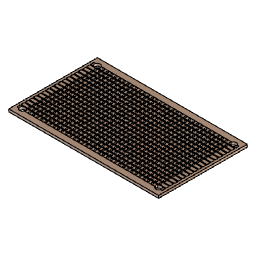
head (Autodesk Fusion 360 archive; units mm, degrees)
design "Veroboard v6"
Autodesk Fusion 360 part; units mm, degrees
sketch "Sketch2" plane through (0, 0, 0) normal (0, 0, 1) x (1, 0, 0) in component "55x93 Tayda Veroboard"
  line L0 (46.5, -27.5) -> (-46.5, -27.5)
  line L1 (-46.5, -27.5) -> (-46.5, 27.5)
  line L2 (-46.5, 27.5) -> (46.5, 27.5)
  line L3 (46.5, 27.5) -> (46.5, -27.5)
  line L4 (46.5, -27.5) -> (-46.5, 27.5) construction
  line L5 (-46.5, -27.5) -> (46.5, 27.5) construction
  line L6 (45, 1) -> (-45, 1)
  line L7 (-45, 1) -> (-45, -1)
  line L8 (-45, -1) -> (45, -1)
  line L9 (45, -1) -> (45, 1)
  line L10 (45, 1) -> (-45, -1) construction
  line L11 (-45, 1) -> (45, -1) construction
  line L12 (45, -21.86) -> (-45, -21.86)
  line L13 (-45, -23.86) -> (45, -23.86)
  line L14 (45, -23.86) -> (45, -21.86)
  line L15 (-45, -21.86) -> (-45, -23.86)
  line L16 (45, -19.32) -> (-45, -19.32)
  line L17 (-45, -21.32) -> (45, -21.32)
  line L18 (45, -21.32) -> (45, -19.32)
  line L19 (-45, -19.32) -> (-45, -21.32)
  line L20 (45, -16.78) -> (-45, -16.78)
  line L21 (-45, -18.78) -> (45, -18.78)
  line L22 (45, -18.78) -> (45, -16.78)
  line L23 (-45, -16.78) -> (-45, -18.78)
  line L24 (45, -14.24) -> (-45, -14.24)
  line L25 (-45, -16.24) -> (45, -16.24)
  line L26 (45, -16.24) -> (45, -14.24)
  line L27 (-45, -14.24) -> (-45, -16.24)
  line L28 (45, -11.7) -> (-45, -11.7)
  line L29 (-45, -13.7) -> (45, -13.7)
  line L30 (45, -13.7) -> (45, -11.7)
  line L31 (-45, -11.7) -> (-45, -13.7)
  line L32 (45, -9.16) -> (-45, -9.16)
  line L33 (-45, -11.16) -> (45, -11.16)
  line L34 (45, -11.16) -> (45, -9.16)
  line L35 (-45, -9.16) -> (-45, -11.16)
  line L36 (45, -6.62) -> (-45, -6.62)
  line L37 (-45, -8.62) -> (45, -8.62)
  line L38 (45, -8.62) -> (45, -6.62)
  line L39 (-45, -6.62) -> (-45, -8.62)
  line L40 (45, -4.08) -> (-45, -4.08)
  line L41 (-45, -6.08) -> (45, -6.08)
  line L42 (45, -6.08) -> (45, -4.08)
  line L43 (-45, -4.08) -> (-45, -6.08)
  line L44 (45, -1.54) -> (-45, -1.54)
  line L45 (-45, -3.54) -> (45, -3.54)
  line L46 (45, -3.54) -> (45, -1.54)
  line L47 (-45, -1.54) -> (-45, -3.54)
  line L48 (45, 3.54) -> (-45, 3.54)
  line L49 (-45, 1.54) -> (45, 1.54)
  line L50 (45, 1.54) -> (45, 3.54)
  line L51 (-45, 3.54) -> (-45, 1.54)
  line L52 (45, 6.08) -> (-45, 6.08)
  line L53 (-45, 4.08) -> (45, 4.08)
  line L54 (45, 4.08) -> (45, 6.08)
  line L55 (-45, 6.08) -> (-45, 4.08)
  line L56 (45, 8.62) -> (-45, 8.62)
  line L57 (-45, 6.62) -> (45, 6.62)
  line L58 (45, 6.62) -> (45, 8.62)
  line L59 (-45, 8.62) -> (-45, 6.62)
  line L60 (45, 11.16) -> (-45, 11.16)
  line L61 (-45, 9.16) -> (45, 9.16)
  line L62 (45, 9.16) -> (45, 11.16)
  line L63 (-45, 11.16) -> (-45, 9.16)
  line L64 (45, 13.7) -> (-45, 13.7)
  line L65 (-45, 11.7) -> (45, 11.7)
  line L66 (45, 11.7) -> (45, 13.7)
  line L67 (-45, 13.7) -> (-45, 11.7)
  line L68 (45, 16.24) -> (-45, 16.24)
  line L69 (-45, 14.24) -> (45, 14.24)
  line L70 (45, 14.24) -> (45, 16.24)
  line L71 (-45, 16.24) -> (-45, 14.24)
  line L72 (45, 18.78) -> (-45, 18.78)
  line L73 (-45, 16.78) -> (45, 16.78)
  line L74 (45, 16.78) -> (45, 18.78)
  line L75 (-45, 18.78) -> (-45, 16.78)
  line L76 (45, 21.32) -> (-45, 21.32)
  line L77 (-45, 19.32) -> (45, 19.32)
  line L78 (45, 19.32) -> (45, 21.32)
  line L79 (-45, 21.32) -> (-45, 19.32)
  line L80 (45, 23.86) -> (-45, 23.86)
  line L81 (-45, 21.86) -> (45, 21.86)
  line L82 (45, 21.86) -> (45, 23.86)
  line L83 (-45, 23.86) -> (-45, 21.86)
  dimension "d17" = 93
  dimension "d18" = 55
  dimension "d19" = 90
  dimension "d20" = 2
  dimension "d23" = 0
  dimension "d24" = 2.54
  constraint horizontal L0
  constraint perpendicular L0 L1
  constraint parallel L0 L2
  constraint parallel L1 L3
  constraint coincident L4 origin
  constraint coincident L5 origin
  constraint horizontal L6
  constraint perpendicular L6 L7
  constraint parallel L6 L8
  constraint parallel L7 L9
  constraint coincident L10 origin
  constraint coincident L11 origin
  measures "d17" distance of L1.end L2.end
  measures "d18" distance of L0.end L1.end
  measures "d19" distance of L7.end L8.end
  measures "d20" distance of L6.end L7.end
extrude "Extrude3" add sketch "Sketch2" against normal blind 1.6 contours L0 L1 L2 L3 | L6 L7 L8 L9 | L12 L13 L14 L15 | L16 L17 L18 L19 | L20 L21 L22 L23 | L24 L25 L26 L27 | L28 L29 L30 L31 | L32 L33 L34 L35 | L36 L37 L38 L39 | L40 L41 L42 L43 | L44 L45 L46 L47 | L48 L49 L50 L51 | L52 L53 L54 L55 | L56 L57 L58 L59 | L60 L61 L62 L63 | L64 L65 L66 L67 | L68 L69 L70 L71 | L72 L73 L74 L75 | L76 L77 L78 L79 | L80 L81 L82 L83 makes body 1 in component "55x93 Tayda Veroboard"
extrude "Extrude4" add sketch "Sketch2" along normal blind 0.05 contours L6 L7 L8 L9 | L12 L13 L14 L15 | L16 L17 L18 L19 | L20 L21 L22 L23 | L24 L25 L26 L27 | L28 L29 L30 L31 | L32 L33 L34 L35 | L36 L37 L38 L39 | L40 L41 L42 L43 | L44 L45 L46 L47 | L48 L49 L50 L51 | L52 L53 L54 L55 | L56 L57 L58 L59 | L60 L61 L62 L63 | L64 L65 L66 L67 | L68 L69 L70 L71 | L72 L73 L74 L75 | L76 L77 L78 L79 | L80 L81 L82 L83 bodies 1 in component "55x93 Tayda Veroboard"
ref_plane "WorkPlane1" through (0, 0, 0.05) normal (0, 0, 1) x (1, 0, 0) in component "55x93 Tayda Veroboard"
sketch "Sketch3" plane through (0, 0, 0.05) normal (0, 0, 1) x (1, 0, 0) in component "55x93 Tayda Veroboard"
  circle A0 centre (0, 0) radius 0.6
  dimension "d33" = 1.2
  constraint coincident A0.centre origin
  measures "d33" diameter of A0
extrude "Extrude5" cut sketch "Sketch3" against normal up to surface (1.65 mm away) bodies 1 in component "55x93 Tayda Veroboard"
pattern_linear "R-Pattern2" count 33 spacing 2.54 along (-1, 0, 0) both ways count 19 spacing 2.54 along (0, -1, 0) both ways of "Extrude5" in component "55x93 Tayda Veroboard"
ref_plane "WorkPlane3" through (0, 0, -1.6) normal (0, 0, -1) x (-1, 0, 0) in component "55x93 Tayda Veroboard"
sketch "Sketch5" plane through (0, 0, -1.6) normal (0, 0, -1) x (1, 0, 0) in component "55x93 Tayda Veroboard"
  circle A0 centre (42.25, 23.25) radius 1.75
  line L0 (46.5, 27.5) -> (-46.5, 27.5)
  line L1 (46.5, -27.5) -> (46.5, 27.5)
  line L2 (0, -1.75) -> (0, -22.5)
  circle A1 centre (-42.25, 23.25) radius 1.75
  line L3 (1.75, 0) -> (22.5, 0)
  circle A2 centre (-42.25, -23.25) radius 1.75
  circle A3 centre (42.25, -23.25) radius 1.75
  dimension "d49" = 3.5
  dimension "d50" = 4.25
  dimension "d51" = 4.25
  constraint symmetric A0 L2 A1
  constraint symmetric A0 L3 A3
  constraint symmetric A1 L3 A2
  measures "d49" diameter of A0
  measures "d50" distance of A0.centre L0
  measures "d51" distance of A0.centre L1
extrude "Extrude6" cut sketch "Sketch5" against normal through all bodies 1 in component "55x93 Tayda Veroboard"
copy_body "CopyPasteBodies1" bodies 1 makes body 2 in component "55x93 Tayda Veroboard"
move_body "Move1" bodies 2 to x (1, 0, 0) y (0, 1, 0) z (0, 0, 1) at (0, 71, 0) in component "55x93 Tayda Veroboard"
copy_body "CutPasteBodies1" bodies 2 removing the originals makes body 3 in component "120x80 Tayda Perf Board"
sketch "Sketch1" plane through (0, 0, 0) normal (0, 0, 1) x (1, 0, 0) in component "120x80 Tayda Perf Board"
  line L0 (40, 60) -> (-40, 60)
  line L1 (-40, 60) -> (-40, -60)
  line L2 (-40, -60) -> (40, -60)
  line L3 (40, -60) -> (40, 60)
  line L4 (40, 60) -> (-40, -60) construction
  line L5 (-40, 60) -> (40, -60) construction
  dimension "d53" = 80
  dimension "d54" = 120
  constraint horizontal L0
  constraint perpendicular L0 L1
  constraint parallel L0 L2
  constraint parallel L1 L3
  constraint coincident L4 origin
  constraint coincident L5 origin
  measures "d53" distance of L1.end L2.end
  measures "d54" distance of L0.end L1.end
extrude "Extrude1" add sketch "Sketch1" against normal blind 1.65 separate body makes body 4 in component "120x80 Tayda Perf Board"
ref_plane "WorkPlane1" through (0, 0, 0) normal (0, 0, 1) x (1, 0, 0) in component "120x80 Tayda Perf Board"
sketch "Sketch2 (2)" plane through (0, 0, 0) normal (0, 0, 1) x (1, 0, 0) in component "120x80 Tayda Perf Board"
  circle A0 centre (0, 0) radius 0.6
  circle A1 centre (0, 0) radius 1
  dimension "d58" = 1.2
  dimension "d59" = 2
  constraint coincident A0.centre A1.centre
  constraint concentric A0 A1
  measures "d58" diameter of A0
  measures "d59" diameter of A1
extrude "Extrude2" cut sketch "Sketch2 (2)" against normal up to surface (1.65 mm away) contours A0 bodies 4 in component "120x80 Tayda Perf Board"
extrude "Extrude3'" add sketch "Sketch2 (2)" along normal blind 0.5 bodies 4 in component "120x80 Tayda Perf Board"
pattern_linear "R-Pattern3" count 29 spacing 2.54 along (-1, 0, 0) both ways count 45 spacing 2.54 along (0, 1, 0) both ways of 1 faces at (0.5993, -0.0299, -0.2167) on bodies 4 in component "120x80 Tayda Perf Board"
pattern_linear "R-Pattern4" count 45 spacing 2.54 along (0, -1, 0) both ways count 29 spacing 2.54 along (-1, 0, 0) both ways of "Extrude3'" in component "120x80 Tayda Perf Board"
ref_plane "WorkPlane2" through (0, 0, 0) normal (0, 0, 1) x (1, 0, 0) in component "120x80 Tayda Perf Board"
sketch "Sketch3 (2)" plane through (0, 0, 0) normal (0, 0, 1) x (1, 0, 0) in component "120x80 Tayda Perf Board"
component "55x93 Tayda Veroboard" placed x (1, 0, 0) y (0, 1, 0) z (0, 0, 1) at (0, 0, 0)
component "Component" placed x (1, 0, 0) y (0, 1, 0) z (0, 0, 1) at (0, 0, 0)
component "120x80 Tayda Perf Board" placed x (1, 0, 0) y (0, 1, 0) z (0, 0, 1) at (0, 0, 0)
hidden bodies 3
